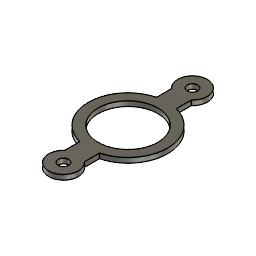
Ring (Autodesk Fusion 360 design; units mm, degrees)
part number: 2026-03-12-21-02-53-361
Autodesk Fusion 360 part; units mm, degrees
sketch "Sketch1" plane through (0, 0, 0) normal (0, 0, 1) x (1, 0, 0)
  circle A0 centre (0, 0) radius 90
  circle A1 centre (0, 65) radius 10
  circle A2 centre (0, -65) radius 10
  circle A3 centre (0, 0) radius 25
  circle A4 centre (0, 0) radius 35
  circle A5 centre (0, 65) radius 20
  circle A6 centre (0, -65) radius 20
  line L0 (-10, 30) -> (10, 30)
  line L1 (10, 30) -> (10, 50)
  line L2 (10, 50) -> (-10, 50)
  line L3 (-10, 50) -> (-10, 30)
  line L4 (-10, -30) -> (10, -30)
  line L5 (10, -30) -> (10, -50)
  line L6 (10, -50) -> (-10, -50)
  line L7 (-10, -50) -> (-10, -30)
  dimension "d1" = 50
  constraint coincident A0.centre A3.centre
  constraint concentric A1 A5
  constraint concentric A2 A6
  constraint horizontal L0
  constraint vertical L1
  constraint horizontal L2
  constraint vertical L3
  constraint horizontal L4
  constraint vertical L5
  constraint horizontal L6
  constraint vertical L7
  measures "d1" diameter of A3
extrude "Extrude1" add sketch "Sketch1" along normal blind 5 contours A4 L0 L1 L3 L4 L5 L7 | A4 L0 L1 L3 | A4 A5 L1 L3 | A4 A6 L5 L7 | A4 L4 L5 L7 | A5 L1 L2 L3 | A5 L1 L2 L3 | A6 L5 L6 L7 | A6 L5 L6 L7 makes body 1
sketch "Sketch2" plane through (0, 0, 0) normal (0, 0, 1) x (1, 0, 0)
sketch "Sketch3" plane through (0, 0, 0) normal (0, 0, 1) x (1, 0, 0)
  circle A0 centre (0, 0) radius 30
  constraint coincident A0.centre origin
extrude "Extrude2" cut sketch "Sketch3" along normal blind 8 bodies 1
sketch "Sketch4" plane through (0, 0, 0) normal (0, 0, 1) x (1, 0, 0)
sketch "Sketch5" plane through (0, 0, 0) normal (0, 1, 0) x (1, 0, 0)
sketch "Sketch6" plane through (0, 0, 0) normal (0, 0, 1) x (1, 0, 0)
  circle A0 centre (0, 65) radius 5.25
  circle A1 centre (0, 65) radius 10
  dimension "d6" = 10.5
  constraint concentric A0 A1
  measures "d6" diameter of A0
extrude "Extrude3" add sketch "Sketch6" along normal blind 5 bodies 1
sketch "Sketch7" plane through (0, 0, 0) normal (0, 0, 1) x (1, 0, 0)
  circle A0 centre (0, -65) radius 5.25
  circle A1 centre (0, -65) radius 10
  dimension "d9" = 10.5
  constraint concentric A0 A1
  measures "d9" diameter of A0
extrude "Extrude4" add sketch "Sketch7" along normal blind 5 bodies 1
sketch "Sketch8" plane through (0, 0, 0) normal (0, 0, 1) x (1, 0, 0)
  circle A0 centre (0, 0) radius 40
  circle A1 centre (0, 0) radius 30
  circle A2 centre (0, 0) radius 30
  constraint coincident A0.centre A1.centre
  constraint concentric A0 A1
  constraint concentric A0 A2
extrude "Extrude5" add sketch "Sketch8" along normal blind 5 bodies 1
sketch "Sketch9" plane through (0, 0, 0) normal (0, 0, 1) x (1, 0, 0)
sketch "Sketch10" plane through (0, 0, 0) normal (0, 0, 1) x (1, 0, 0)
sketch "Sketch11" plane through (0, 0, 0) normal (0, 0, 1) x (1, 0, 0)
sketch "Sketch12" plane through (0, 0, 0) normal (0, 0, 1) x (1, 0, 0)
  circle A0 centre (0, 65) radius 15
  circle A1 centre (0, 65) radius 20
  constraint concentric A0 A1
extrude "Extrude6" cut sketch "Sketch12" along normal blind 30 bodies 1 makes body 2 at (11.6746, 63.994, 0)
sketch "Sketch13" plane through (0, 0, 0) normal (0, 0, 1) x (1, 0, 0)
  circle A0 centre (0, -65) radius 15
  circle A1 centre (0, -65) radius 20
  constraint concentric A0 A1
extrude "Extrude7" cut sketch "Sketch13" along normal blind 22 bodies 1 makes body 3 at (3.3287, -53.7649, 0)
sketch "Sketch14" plane through (0, 0, 0) normal (0, 0, 1) x (1, 0, 0)
  line L0 (-10, -35) -> (10, -35)
  line L1 (10, -35) -> (10, -59)
  line L2 (10, -59) -> (-10, -59)
  line L3 (-10, -59) -> (-10, -35)
  line L4 (-10, 35) -> (10, 35)
  line L5 (10, 35) -> (10, 58)
  line L6 (10, 58) -> (-10, 58)
  line L7 (-10, 58) -> (-10, 35)
  constraint horizontal L0
  constraint vertical L1
  constraint horizontal L2
  constraint vertical L3
  constraint horizontal L4
  constraint vertical L5
  constraint horizontal L6
  constraint vertical L7
extrude "Extrude8" add sketch "Sketch14" along normal blind 5 bodies 1 2 3
